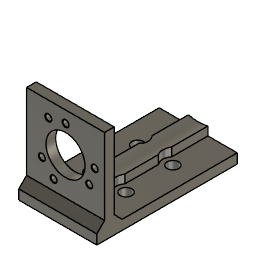
Base_encoder (Autodesk Fusion 360 design; units mm, degrees)
Autodesk Fusion 360 part; units mm, degrees
sketch "Sketch1" plane through (0, 0, 0) normal (0, 0, 1) x (1, 0, 0)
  line L0 (0, 0) -> (30, 0)
  line L1 (30, 0) -> (30, 34)
  line L2 (30, 34) -> (0, 34)
  line L3 (0, 34) -> (0, 0)
  line L4 (0, 17) -> (30, 17) construction
  line L5 (15, 34) -> (15, 17) construction
  line L6 (15, 17) -> (15, 5) construction
  line L7 (15, 5) -> (6, 5)
  circle A0 centre (6, 5) radius 2.05
  circle A1 centre (6, 5) radius 3
  circle A2 centre (24, 5) radius 3
  circle A3 centre (24, 5) radius 2.05
  circle A4 centre (24, 29) radius 3
  circle A5 centre (24, 29) radius 2.05
  circle A6 centre (6, 29) radius 3
  circle A7 centre (6, 29) radius 2.05
  line L8 (35, -21) -> (-5, -21)
  line L9 (-5, -21) -> (-5, 55)
  line L10 (-5, 55) -> (35, 55)
  line L11 (35, 55) -> (35, -21)
  line L12 (35, -21) -> (-5, 55) construction
  line L13 (-5, -21) -> (35, 55) construction
  line L14 (35, -17) -> (-5, -17)
  line L15 (-5, -17) -> (-5, 51)
  line L16 (-5, 51) -> (35, 51)
  line L17 (35, 51) -> (35, -17)
  line L18 (35, -17) -> (-5, 51) construction
  line L19 (-5, -17) -> (35, 51) construction
  line L20 (-5, -12) -> (35, -12)
  line L21 (35, -12) -> (35, -17)
  line L22 (35, -17) -> (-5, -17)
  line L23 (-5, -17) -> (-5, -12)
  point P0 (15, 17)
  point P1 (15, 17)
  dimension "d1" = 34
  dimension "d2" = 30
  dimension "d3" = 12
  dimension "d4" = 9
  dimension "d5" = 4.1
  dimension "d6" = 6
  dimension "d7" = 76
  dimension "d8" = 68
  dimension "d48" = 5
  dimension "d53" = 40
  constraint horizontal L0
  constraint vertical L1
  constraint horizontal L2
  constraint vertical L3
  constraint coincident L0.start L3.end
  constraint midpoint L3 L4.start
  constraint midpoint L1 L4.end
  constraint midpoint L2 L5.start
  constraint midpoint L4 P1
  constraint perpendicular L4 L6
  constraint perpendicular L6 L7
  constraint coincident L7.end A0.centre
  constraint concentric A0 A1
  constraint symmetric L6 A0 A3
  constraint symmetric L6 A1 A2
  constraint symmetric L4 A0 A7
  constraint symmetric L4 A1 A6
  constraint symmetric L4 A2 A4
  constraint symmetric L4 A3 A5
  constraint horizontal L8
  constraint perpendicular L8 L9
  constraint parallel L8 L10
  constraint parallel L9 L11
  constraint coincident L12 P1
  constraint coincident L13 P1
  constraint coincident P1 P0
  constraint horizontal L14
  constraint perpendicular L14 L15
  constraint parallel L14 L16
  constraint parallel L15 L17
  constraint coincident L18 P1
  constraint coincident L19 P1
  constraint horizontal L20
  constraint vertical L21
  constraint horizontal L22
  constraint vertical L23
  constraint coincident L15 L20.start
  constraint coincident L9 L20.start
  measures "d1" distance of L0 L2
  measures "d2" distance of L1 L3
  measures "d3" distance of P1 L6.end
  measures "d4" distance of L6.end L7.end
  measures "d5" diameter of A0
  measures "d6" diameter of A1
  measures "d7" distance of L8.end L9.end
  measures "d8" distance of L14.end L15.end
  measures "d48" distance of L14 L20
  measures "d53" distance of L9.end L10.end
extrude "Extrude1" add sketch "Sketch1" along normal blind 2 contours L0 L1 L2 L3 | L8 L9 L11 L14 L22 | L9 L11 L15 L16 L17 L20 makes body 1 at (21.6667, -19.6667, 0) makes body 2 at (12.3653, 44.5975, 0)
extrude "Extrude2" add sketch "Sketch1" along normal blind 45 contours L9 L11 L14 L15 L17 L20 L21 L22 L23 bodies 1 2
sketch "Sketch2" plane through (0, -17, 0) normal (0, -1, 0) x (1, 0, 0)
  line L0 (-5, 2) -> (35, 2)
  line L1 (35, 2) -> (35, 45)
  line L2 (35, 45) -> (-5, 45)
  line L3 (-5, 45) -> (-5, 2)
  circle A0 centre (15, 25) radius 19 construction
  circle A1 centre (15, 25) radius 14 construction
  circle A2 centre (15, 25) radius 15 construction
  circle A3 centre (15, 39) radius 1.55
  line L4 (15, 25) -> (15, 39) construction
  line L5 (15, 25) -> (6.1832, 37.1353) construction
  circle A4 centre (6.1832, 37.1353) radius 1.55
  circle A5 centre (2.8756, 18) radius 1.55
  circle A6 centre (27.1244, 18) radius 1.55
  circle A7 centre (8.899, 11.2968) radius 1.55
  circle A8 centre (29.9178, 26.5679) radius 1.55
  circle A9 centre (15, 25) radius 10
  dimension "d14" = 38
  dimension "d15" = 28
  dimension "d16" = 30
  dimension "d17" = 3.1
  dimension "d20" = 36
  dimension "d21" = 3.1
  dimension "d23" = 360
  dimension "d25" = 360
  dimension "d30" = 20
  dimension "d31" = 20
  constraint concentric A0 A1
  constraint concentric A1 A2
  constraint coincident A0.centre A1.centre
  constraint coincident A3.centre L4.end
  constraint vertical L4
  constraint coincident A2 L5.end
  constraint coincident L5.end A4.centre
  constraint concentric A0 A9
  measures "d14" diameter of A0
  measures "d15" diameter of A1
  measures "d16" diameter of A2
  measures "d17" diameter of A3
  measures "d20" angle of L4 L5
  measures "d21" diameter of A4
  measures "d30" diameter of A9
  measures "d31" distance of L2 A0.centre
extrude "Extrude3" cut sketch "Sketch2" against normal blind 6 contours A3 | A4 | A5 | A6 | A7 | A8 | A9 bodies 1
fillet "Fillet1" radius 0.2 6 edges at (4.7381, -17, 37.6958) (13.5549, -17, 39.5605) (28.4727, -17, 27.1284) (25.6792, -17, 18.5605) (7.4538, -17, 11.8573) (1.4305, -17, 18.5605) on bodies 1
sketch "Sketch3" plane through (0, 51, 0) normal (0, 1, 0) x (-1, 0, 0)
  line L0 (-35, 0) -> (5, 0)
  line L1 (5, 0) -> (5, 2)
  line L2 (5, 2) -> (-35, 2)
  line L3 (-35, 2) -> (-35, 0)
  line L4 (-35, 45) -> (5, 45)
  line L5 (5, 45) -> (5, 3)
  line L6 (5, 3) -> (-35, 3)
  line L7 (-35, 3) -> (-35, 45)
  circle A0 centre (-15, 25) radius 19
  line L8 (-35, 3) -> (-20, 3)
  line L9 (5, 3) -> (-10, 3)
  line L10 (-20, 3) -> (-20, 6.4202)
  line L11 (-10, 3) -> (-10, 6.42)
  arc A1 (-20, 6.4202) -> (-10, 6.42) centre (-14.9996, 24.8774) ccw
  line L12 (-20, 3) -> (-10, 3)
  line L13 (-10, 3) -> (-10, 2)
  line L14 (-10, 2) -> (-20, 2)
  line L15 (-20, 2) -> (-20, 3)
  dimension "d42" = 38
  dimension "d43" = 15
  dimension "d44" = 15
  dimension "d45" = 3.42
  constraint horizontal L4
  constraint vertical L5
  constraint horizontal L6
  constraint vertical L7
  constraint perpendicular L7 L8
  constraint perpendicular L5 L9
  constraint perpendicular L6 L10
  constraint perpendicular L6 L11
  constraint tangent A0 A1
  constraint horizontal L12
  constraint vertical L13
  constraint horizontal L14
  constraint vertical L15
  constraint coincident L2 L13.end
  measures "d42" diameter of A0
  measures "d43" distance of L6.end L8.end
  measures "d44" distance of L5.end L9.end
  measures "d45" distance of L9.end L11.end
extrude "Extrude4" add sketch "Sketch3" against normal up to surface (63 mm away) contours L2 L6 L12 L13 L14 L15 | L6 L10 L11 A1 L12 bodies 1
chamfer "Chamfer3" distance 4 angle 45 1 edges at (15, -17, 2) on bodies 1
chamfer "Chamfer4" distance 4 angle 45 2 edges at (2.5, -12, 2) (27.5, -12, 2) on bodies 1
extrude "Extrude5" add 1 faces at (17.6347, -13.2642, 0) along direction (0, 0, -1) blind 3 on bodies 1 bodies 1
sketch "Boceto4" plane through (0, 0, 2) normal (0, 0, 1) x (-1, 0, 0)
  line L0 (-20, 8) -> (-35, 8)
  line L1 (-35, 8) -> (-35, -51)
  line L2 (-35, -51) -> (-20, -51)
  line L3 (-20, -51) -> (-20, 8)
  line L4 (-10, 8) -> (-10, -51)
  line L5 (-10, -51) -> (5, -51)
  line L6 (5, -51) -> (5, 8)
  circle A0 centre (-6, -29) radius 3
  circle A1 centre (-24, -29) radius 3
  circle A2 centre (-24, -5) radius 3
  circle A3 centre (-6, -5) radius 3
  circle A4 centre (-24, -5) radius 5.25
  circle A5 centre (-24, -29) radius 5.25
  circle A6 centre (-6, -29) radius 5.25
  circle A7 centre (-6, -5) radius 5.25
  line L7 (5, 8) -> (-10, 8)
  dimension "d54" = 10.5
  dimension "d55" = 10.5
  dimension "d56" = 10.5
  dimension "d57" = 10.5
  constraint concentric A2 A4
  constraint concentric A1 A5
  constraint concentric A0 A6
  constraint concentric A3 A7
  measures "d54" diameter of A4
  measures "d55" diameter of A5
  measures "d56" diameter of A6
  measures "d57" diameter of A7
extrude "Extruir6" cut sketch "Boceto4" along normal blind 5 contours L3 A4 | L3 A5 | L4 A7 | L4 A6 picked at (-19.3381, -4.8303) picked at (-19.854, -29.935) picked at (-10.4167, -5) picked at (-10.4167, -29) bodies 1
equation "d7 = 78 mm - 2 mm"
equation "d8 = 70 mm - 2 mm"
